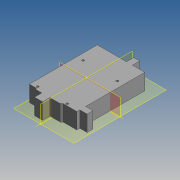
# Autodesk Inventor part: P016_FondBoitierCapteurs
Saved by Autodesk Inventor 2021.3 (Build 253353000, 353)
## iProperties
Created: 2021-10-29
Part Number: P016_FondBoitierCapteurs
Material: Générique
Document SubType Name: Modeling
Designer: gabri
Density: 1 g/cm^3
Appearance: Par défaut
Author: gabri
Autodesk Inventor part; units mm, degrees
sketch "Sketch2" plane through (0, 0, 0) normal (0, 0, 1) x (1, 0, 0)
  line L0 (11.535, -47.52) -> (-21.535, -47.52)
  line L1 (-32.535, -45.52) -> (-32.535, 47.52)
  line L2 (-32.535, 47.52) -> (32.535, 47.52)
  line L3 (32.535, 47.52) -> (32.535, -45.52)
  line L4 (32.535, -47.52) -> (-32.535, 47.52) construction
  line L5 (-32.535, -47.52) -> (32.535, 47.52) construction
  line L6 (-32.535, -45.52) -> (-23.535, -45.52)
  line L7 (-23.535, -45.52) -> (-21.535, -47.52)
  line L8 (11.535, -47.52) -> (13.535, -45.52)
  line L9 (13.535, -45.52) -> (32.535, -45.52)
  circle A0 centre (-23.985, -42.97) radius 1.55
  circle A1 centre (16.585, -42.97) radius 1.55
  circle A2 centre (-23.985, 19.39) radius 1.55
  circle A3 centre (23.985, 18.43) radius 1.55
  line L10 (-47.549, 0) -> (57.549, 0) construction
  line L11 (0, 80.528) -> (0, -80.528) construction
  line L12 (-13.535, -47.52) -> (-2.535, -47.52)
  line L13 (-2.535, -47.52) -> (-2.535, -57.52)
  line L14 (-2.535, -57.52) -> (-13.535, -57.52)
  line L15 (-13.535, -57.52) -> (-13.535, -47.52)
  line L16 (32.535, -33.52) -> (42.535, -33.52)
  line L17 (42.535, -33.52) -> (42.535, -41.52)
  line L18 (42.535, -41.52) -> (32.535, -41.52)
  line L19 (32.535, -41.52) -> (32.535, -33.52)
  line L20 (7.535, 47.52) -> (15.535, 47.52)
  line L21 (15.535, 47.52) -> (15.535, 57.52)
  line L22 (15.535, 57.52) -> (7.535, 57.52)
  line L23 (7.535, 57.52) -> (7.535, 47.52)
  point P0 (0, 0)
  point P1 (0, 0)
  point P2 (0, 0)
  dimension "d56" = 65.07
  dimension "d57" = 95.04
  dimension "d58" = 2
  dimension "d59" = 9
  dimension "d60" = 11
  dimension "d61" = 21
  dimension "d62" = 19
  dimension "d63" = 8.55
  dimension "d64" = 3.1
  dimension "d65" = 2.55
  dimension "d66" = 2.55
  dimension "d67" = 15.95
  dimension "d68" = 8.55
  dimension "d69" = 64.91
  dimension "d70" = 3.1
  dimension "d71" = 3.1
  dimension "d72" = 3.1
  dimension "d73" = 63.95
  dimension "d74" = 8.55
  dimension "d75" = 47.52
  dimension "d76" = 32.535
  dimension "d77" = 19
  dimension "d78" = 11
  dimension "d79" = 10
  dimension "d80" = 4
  dimension "d81" = 8
  dimension "d82" = 10
  dimension "d83" = 8
  dimension "d84" = 10
  dimension "d85" = 17
  constraints: 44 end point, 8 parallel, 5 perpendicular, 5 point on line, 4 centre point, 4 horizontal, 3 midpoint, 1 coincident
  measures "d56" distance of L1.end L2.end
  measures "d57" distance between parallel lines of L0 L2
  measures "d58" distance between parallel lines of L0 L6
  measures "d59" distance of L1.start L6.end
  measures "d60" distance from line of L0.end L1
  measures "d61" distance from line of L0.start L3
  measures "d62" distance from line of L3 L8.end
  measures "d63" distance from line of A0.centre L1
  measures "d64" diameter of A0
  measures "d65" distance from line of L6 A0.centre
  measures "d66" distance from line of L9 A1.centre
  measures "d67" distance from line of L3 A1.centre
  measures "d68" distance from line of L1 A2.centre
  measures "d69" distance from line of L6 A2.centre
  measures "d70" diameter of A2
  measures "d71" diameter of A1
  measures "d72" diameter of A3
  measures "d73" distance from line of L9 A3.centre
  measures "d74" distance from line of L3 A3.centre
  measures "d75" distance between parallel lines of L10 L2
  measures "d76" distance between parallel lines of L11 L1
  measures "d77" distance between parallel lines of L15 L1
  measures "d78" distance between parallel lines of L13 L15
  measures "d79" distance between parallel lines of L14 L0
  measures "d80" distance between parallel lines of L18 L9
  measures "d81" distance between parallel lines of L18 L16
  measures "d82" distance of L16.start L16.end
  measures "d83" distance between parallel lines of L21 L23
  measures "d84" distance between parallel lines of L20 L22
  measures "d85" distance between parallel lines of L3 L21
extrude "Extrusion1" add sketch "Sketch2" along normal blind 22
equation "\"d66\" = d65"
body "Solid1"
